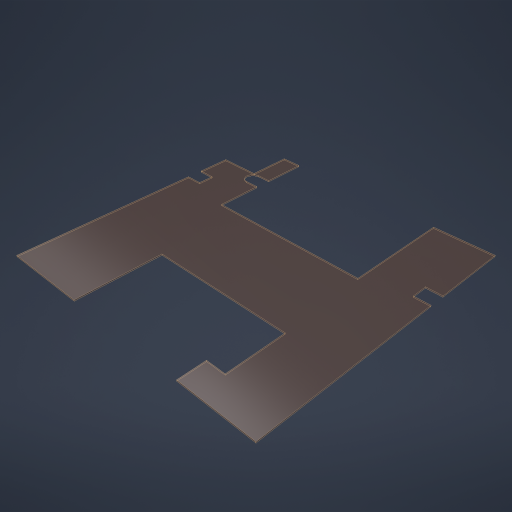
# Autodesk Inventor part: DB1-023
Saved by Autodesk Inventor 2023.4 (Build 274418000, 418)
## iProperties
Created: 2025-03-10
Part Number: DB1-023
Material: Polycarbonate, Smoke
Document SubType Name: Sheet Metal
Designer: brand
Density: 1.2 g/cm^3
Sheet Metal Rule: Default
Appearance: Polycarbonate - Smoked
Author: brand
Autodesk Inventor part; units mm, degrees
ref_plane "YZ Plane" through (0, 0, 0) normal (1, 0, 0) x (0, 1, 0)
ref_plane "XZ Plane" through (0, 0, 0) normal (0, 1, 0) x (-1, 0, 0)
ref_plane "XY Plane" through (0, 0, 0) normal (0, 0, 1) x (1, 0, 0)
sketch "Sketch1" plane through (0, 0, 0) normal (0, 1, 0) x (-1, 0, 0)
  line L0 (329.819, 329.819) -> (-329.819, 329.819)
  line L1 (-329.819, 329.819) -> (-329.819, -329.819)
  line L2 (-329.819, -329.819) -> (329.819, -329.819)
  line L3 (329.819, -329.819) -> (329.819, 329.819)
  line L4 (329.819, 329.819) -> (-329.819, -329.819) construction
  line L5 (-329.819, 329.819) -> (329.819, -329.819) construction
  line L6 (133.35, 329.819) -> (-133.35, 329.819) construction
  line L7 (-133.35, 329.819) -> (-133.35, 126.619)
  line L8 (-133.35, 126.619) -> (133.35, 126.619)
  line L9 (133.35, 126.619) -> (133.35, 329.819)
  line L10 (187.325, -329.819) -> (-187.325, -329.819) construction
  line L11 (-187.325, -329.819) -> (-187.325, -82.169)
  line L12 (-187.325, -82.169) -> (187.325, -82.169)
  line L13 (187.325, -82.169) -> (187.325, -329.819)
  point P0 (0, 0)
  point P1 (0, 329.819)
  point P2 (0, 329.819)
  point P3 (0, -329.819)
  point P4 (0, -329.819)
  point P5 (-133.35, 329.819)
  dimension "d0" = 659.638
  dimension "d1" = 659.638
  dimension "d2" = 266.7
  dimension "d3" = 203.2
  dimension "d4" = 247.65
  dimension "d5" = 374.65
  constraints: 28 end point, 6 midpoint, 6 parallel, 3 horizontal, 3 perpendicular, 2 coincident, 2 point on line
  measures "d0" distance of L0.start L0.end
  measures "d1" distance of L2.end L0.start
  measures "d2" distance of L7.end L8.end
  measures "d3" distance of L8.end L6.start
  measures "d4" distance of L12.end L10.start
  measures "d5" distance of L11.end L12.end
extrude "Extrusion1" add sketch "Sketch1" along normal mid plane 3.175 contours L3 L2 L13 L12 L11 L1 L0 L7 L8 L9
sketch "Sketch2" plane through (0, 1.5875, 0) normal (0, 1, 0) x (1, 0, 0)
  circle A0 centre (-283.3124, 275.8316) radius 34.925 construction
  line L0 (329.819, 329.819) -> (329.819, -329.819) construction
  line L1 (329.819, -329.819) -> (133.35, -329.819) construction
  line L2 (133.35, -329.819) -> (133.35, -126.619) construction
  line L3 (133.35, -126.619) -> (-133.35, -126.619) construction
  line L4 (-133.35, -126.619) -> (-133.35, -329.819) construction
  line L5 (-133.35, -329.819) -> (-329.819, -329.819) construction
  line L6 (-329.819, -329.819) -> (-329.819, 329.819) construction
  line L7 (-329.819, 329.819) -> (-187.325, 329.819) construction
  line L8 (-187.325, 329.819) -> (-187.325, 82.169) construction
  line L9 (-187.325, 82.169) -> (187.325, 82.169) construction
  line L10 (187.325, 82.169) -> (187.325, 329.819) construction
  line L11 (187.325, 329.819) -> (329.819, 329.819) construction
  line L12 (-187.325, 329.819) -> (-329.819, 329.819) construction
  line L13 (-329.819, 329.819) -> (-234.569, 329.819)
  line L14 (-234.569, 329.819) -> (-234.569, 228.219)
  line L15 (-234.569, 228.219) -> (-329.819, 228.219)
  line L16 (-329.819, 228.219) -> (-329.819, 329.819)
  line L17 (329.819, -329.819) -> (133.35, -329.819) construction
  line L18 (133.35, -126.619) -> (152.4, -126.619)
  line L19 (152.4, -126.619) -> (152.4, -329.819)
  line L20 (152.4, -329.819) -> (133.35, -329.819)
  line L21 (133.35, -329.819) -> (133.35, -126.619)
  line L22 (-329.819, 329.819) -> (-329.819, -329.819) construction
  line L23 (-329.819, 149.606) -> (-291.719, 149.606)
  line L24 (-291.719, 149.606) -> (-291.719, 111.506)
  line L25 (-291.719, 111.506) -> (-329.819, 111.506)
  line L26 (-329.819, 111.506) -> (-329.819, 149.606)
  line L27 (329.819, 149.606) -> (291.719, 149.606)
  line L28 (291.719, 149.606) -> (291.719, 111.506)
  line L29 (291.719, 111.506) -> (329.819, 111.506)
  line L30 (329.819, 111.506) -> (329.819, 149.606)
  line L31 (152.4, -126.619) -> (196.85, -126.619)
  line L32 (196.85, -126.619) -> (196.85, -266.319)
  line L33 (196.85, -266.319) -> (152.4, -266.319)
  line L34 (152.4, -266.319) -> (152.4, -126.619)
  point P0 (0, 0)
  point P1 (-329.819, 130.556)
  point P2 (152.4, -266.319)
  dimension "d9" = 69.85
  dimension "d10" = 46.5066
  dimension "d11" = 53.9874
  dimension "d12" = 101.6
  dimension "d13" = 95.25
  dimension "d16" = 19.05
  dimension "d17" = 460.375
  dimension "d18" = 38.1
  dimension "d19" = 38.1
  dimension "d20" = 63.5
  dimension "d21" = 63.5
  constraints: 40 end point, 11 parallel, 5 horizontal, 5 perpendicular, 3 point on line, 2 horizontal alignment, 1 centre point, 1 midpoint
  measures "d9" diameter of A0
  measures "d10" distance from line of L16 A0.centre
  measures "d11" distance from line of L7 A0.centre
  measures "d12" distance of L13.end L14.end
  measures "d13" distance of L14.end L15.end
  measures "d16" distance of L2.end L18.end
  measures "d17" distance from line of L5 point (-329.819, 130.556)
  measures "d18" distance of L23.end L24.end
  measures "d19" distance of L24.end L25.end
  measures "d20" distance between parallel lines of L2 L32
  measures "d21" distance between parallel lines of L1 L33
extrude "Extrusion2" cut sketch "Sketch2" against normal through all
sketch "Sketch3" plane through (0, 1.5875, 0) normal (0, 1, 0) x (1, 0, 0)
  line L0 (-291.719, 111.506) -> (-291.719, 149.606) construction
  line L1 (-291.719, 149.606) -> (-329.819, 149.606) construction
  line L2 (-329.819, 149.606) -> (-329.819, 228.219) construction
  line L3 (-329.819, 228.219) -> (-234.569, 228.219) construction
  line L4 (-234.569, 228.219) -> (-234.569, 329.819) construction
  line L5 (-234.569, 329.819) -> (-187.325, 329.819) construction
  line L6 (-187.325, 329.819) -> (-187.325, 82.169) projected
  line L7 (-187.325, 82.169) -> (187.325, 82.169) construction
  line L8 (187.325, 82.169) -> (187.325, 329.819) construction
  line L9 (187.325, 329.819) -> (329.819, 329.819) construction
  line L10 (329.819, 329.819) -> (329.819, 149.606) construction
  line L11 (329.819, 149.606) -> (291.719, 149.606) construction
  line L12 (291.719, 149.606) -> (291.719, 111.506) construction
  line L13 (291.719, 111.506) -> (329.819, 111.506) construction
  line L14 (329.819, 111.506) -> (329.819, -329.819) construction
  line L15 (329.819, -329.819) -> (152.4, -329.819) construction
  line L16 (152.4, -329.819) -> (152.4, -266.319) construction
  line L17 (152.4, -266.319) -> (196.85, -266.319) construction
  line L18 (196.85, -266.319) -> (196.85, -126.619) construction
  line L19 (196.85, -126.619) -> (-133.35, -126.619) construction
  line L20 (-133.35, -126.619) -> (-133.35, -329.819) construction
  line L21 (-133.35, -329.819) -> (-329.819, -329.819) construction
  line L22 (-329.819, -329.819) -> (-329.819, 111.506) construction
  line L23 (-329.819, 111.506) -> (-291.719, 111.506) construction
  circle A0 centre (-219.075, 209.169) radius 19.05
  line L24 (-219.075, 228.219) -> (-187.325, 228.219)
  line L25 (-187.325, 82.169) -> (-187.325, 329.819) construction
  line L26 (-219.075, 190.119) -> (-187.325, 190.119)
  point P0 (0, 0)
  dimension "d22" = 38.1
  dimension "d23" = 120.65
  dimension "d24" = 31.75
  constraints: 4 end point, 2 perpendicular, 2 point on circle, 2 point on line, 2 tangent, 1 centre point
  measures "d22" diameter of A0
  measures "d23" distance from line of L5 A0.centre
  measures "d24" distance from line of L6 A0.centre
extrude "Extrusion3" cut sketch "Sketch3" against normal through all
equation "\"d19\" = d18"
equation "\"BendRadius\" = Thickness"
equation "\"BendReliefWidth\" = Thickness"
equation "\"BendReliefDepth\" = 0.5 * Thickness"
equation "\"CornerReliefSize\" = 4 * Thickness"
equation "\"MinimumRemnant\" = 2 * Thickness"
equation "\"TransitionRadius\" = BendRadius"
equation "\"JacobiRadiusSize\" = BendRadius"
equation "\"GapSize\" = Thickness"
equation "\"Thickness\" = 3.048"
body "Solid1"
